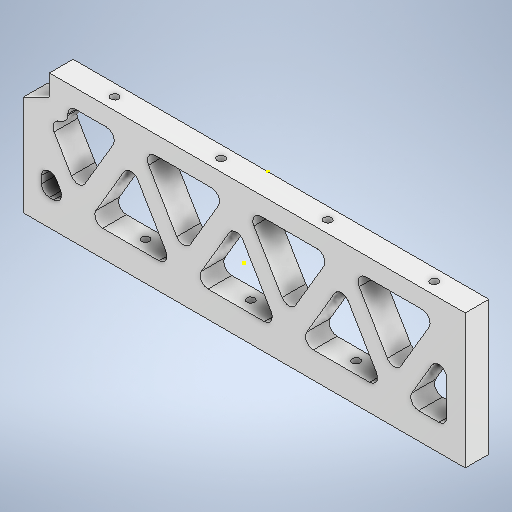
# Autodesk Inventor part: RightTruss
Saved by Autodesk Inventor 2026.2 (Build 302298000, 298)
## iProperties
Created: 2026-04-01
Part Number: RightTruss
Material: ABS Plastic
Document SubType Name: Modeling
Designer: gaoet
Density: 1.06 g/cm^3
Appearance: Smooth - White
Author: gaoet
Autodesk Inventor part; units mm, degrees
ref_plane "YZ Plane" through (0, 0, 0) normal (1, 0, 0) x (0, 1, 0)
ref_plane "XZ Plane" through (0, 0, 0) normal (0, 1, 0) x (-1, 0, 0)
ref_plane "XY Plane" through (0, 0, 0) normal (0, 0, 1) x (1, 0, 0)
sketch "Sketch1" plane through (0, 0, 0) normal (0, 0, 1) x (1, 0, 0)
  line L0 (-84, -25.5) -> (84, -25.5)
  line L1 (84, -25.5) -> (84, 25.5)
  line L2 (84, 25.5) -> (-84, 25.5)
  line L3 (-84, 25.5) -> (-84, -25.5)
  line L4 (-84, -25.5) -> (84, 25.5) construction
  line L5 (84, -25.5) -> (-84, 25.5) construction
  line L6 (-84, 17.5) -> (-74, 17.5)
  line L7 (-74, 17.5) -> (-74, 25.5)
  point P0 (0, 0)
  dimension "d0" = 168
  dimension "d1" = 51
  dimension "d2" = 10
  dimension "d3" = 8
  constraints: 16 end point, 2 horizontal, 2 midpoint, 2 parallel, 2 perpendicular, 2 point on line
  measures "d0" distance of L2.end L1.end
  measures "d1" distance of L0.end L1.end
  measures "d2" distance of L6.start L6.end
  measures "d3" distance of L6.end L7.end
extrude "Extrusion1" add sketch "Sketch1" along normal blind 9 contours L3 L6 L7 L2 L1 L0
chamfer "Chamfer1" distance 10 distance2 5 1 edges at (-84, 17.5, 4.5) measured on face at (-77.3333, 17.5, 3)
sketch "Sketch2" plane through (-84, -25.5, 0) normal (0, -1, 0) x (1, 0, 0)
  line L0 (0, 0) -> (0, 9) projected
  line L1 (0, 0) -> (168, 0) projected
  point P0 (84, 0)
  point P1 (22, 4.5)
  point P2 (42, 4.5)
  point P3 (62, 4.5)
  point P4 (82, 4.5)
  point P5 (102, 4.5)
  point P6 (122, 4.5)
  point P7 (142, 4.5)
  point P8 (162, 4.5)
  dimension "d9" = 22
  dimension "d10" = 4.5
  dimension "d13" = 20
  constraints: 1 horizontal, 7 other
  measures "d9" distance from line of L0 point (22, 4.5)
  measures "d10" distance from line of L1 point (22, 4.5)
  measures "d13" distance of point (22, 4.5) point (42, 4.5)
hole "Hole1" at (-62, -25.5, 4.5) at (-42, -25.5, 4.5) at (-22, -25.5, 4.5) at (-2, -25.5, 4.5) at (18, -25.5, 4.5) at (38, -25.5, 4.5) at (58, -25.5, 4.5) direction (0, 1, 0) diameter 3 depth 10
sketch "Sketch3" plane through (0, 0, 9) normal (0, 0, 1) x (1, 0, 0)
  line L0 (-63.5, -15.5) -> (-60.5, -15.5) projected
  line L1 (-84, 12.5) -> (-84, -25.5) projected
  line L2 (-84, -15.5) -> (84, -15.5)
  line L3 (84, -25.5) -> (84, 25.5) projected
  line L4 (-84, 12.5) -> (-74, 17.5) projected
  line L5 (-84, 12.5) -> (-84, -25.5) projected
  line L6 (-84, -25.5) -> (84, -25.5) projected
  line L7 (84, -25.5) -> (84, 25.5) projected
  line L8 (84, 25.5) -> (-74, 25.5) projected
  line L9 (-74, 25.5) -> (-74, 17.5) projected
  line L10 (-67, 18.5) -> (77, 18.5)
  line L11 (77, 18.5) -> (77, -18.5)
  line L12 (77, -18.5) -> (-77, -18.5)
  line L13 (-77, -18.5) -> (-77, 8.1738)
  line L14 (-77, 8.1738) -> (-67, 13.1738)
  line L15 (-67, 13.1738) -> (-67, 18.5)
  line L16 (77, 18.5) -> (56.9904, -15.5) construction
  line L17 (36.9807, 18.5) -> (56.9904, -15.5) construction
  line L18 (16.9711, -15.5) -> (36.9807, 18.5) construction
  line L19 (-3.0386, 18.5) -> (16.9711, -15.5) construction
  line L20 (-23.0482, -15.5) -> (-3.0386, 18.5) construction
  line L21 (-23.0482, -15.5) -> (-43.0579, 18.5) construction
  line L22 (-63.0675, -15.5) -> (-43.0579, 18.5) construction
  line L23 (-77, 8.1738) -> (-63.0675, -15.5) construction
  line L24 (-63.5, -15.5) -> (-60.5, -15.5) projected
  line L25 (-63.0675, -15.5) -> (-83.0772, 18.5) construction
  line L26 (-77, 1.2732) -> (-67.1287, -15.5)
  line L27 (-73.8622, 9.7427) -> (-59.0064, -15.5)
  line L28 (-47.119, 18.5) -> (-67.1287, -15.5)
  line L29 (-38.9968, 18.5) -> (-59.0064, -15.5)
  line L30 (-47.119, 18.5) -> (-27.1094, -15.5)
  line L31 (-38.9968, 18.5) -> (-18.9871, -15.5)
  line L32 (-7.0997, 18.5) -> (-27.1094, -15.5)
  line L33 (-18.9871, -15.5) -> (1.0225, 18.5)
  line L34 (-7.0997, 18.5) -> (12.9099, -15.5)
  line L35 (1.0225, 18.5) -> (21.0322, -15.5)
  line L36 (12.9099, -15.5) -> (32.9196, 18.5)
  line L37 (41.0418, 18.5) -> (61.0515, -15.5)
  line L38 (77, 11.5994) -> (61.0515, -15.5)
  line L39 (32.9196, 18.5) -> (52.9292, -15.5)
  line L40 (41.0418, 18.5) -> (21.0322, -15.5)
  line L41 (72.9389, 18.5) -> (52.9292, -15.5)
  point P0 (0, 0)
  point P1 (-73.0724, 1.5)
  point P2 (-72.0643, -7.1134)
  point P3 (26.9759, 1.5)
  point P4 (77, -15.5)
  point P5 (-3.0386, 11.5994)
  point P6 (56.9904, -8.5994)
  point P7 (36.9807, 11.5994)
  point P8 (16.9711, -8.5994)
  point P9 (-23.0482, -8.5994)
  point P10 (-43.0579, 11.5994)
  point P11 (-77, -15.5)
  point P12 (-63.0675, -8.5994)
  dimension "d25" = 7
  dimension "d30" = 3.5
  dimension "d31" = 3.5
  dimension "d32" = 3.5
  dimension "d33" = 3.5
  dimension "d34" = 3.5
  dimension "d35" = 3.5
  dimension "d36" = 3.5
  dimension "d37" = 3.5
  dimension "d38" = 3.5
  dimension "d39" = 3.5
  dimension "d40" = 3.5
  dimension "d41" = 3.5
  dimension "d42" = 3.5
  dimension "d43" = 3.5
  dimension "d44" = 3.5
  dimension "d46" = 3.5
  constraints: 60 end point, 16 parallel, 7 equal length, 7 point on line, 3 midpoint, 1 collinear, 1 horizontal, 1 horizontal alignment, 47 other
  measures "d30" distance from line of point (-73.072, 1.5) L27
  measures "d31" distance from line of point (-72.064, -7.113) L23
  measures "d32" distance between parallel lines of L22 L28
  measures "d33" distance between parallel lines of L29 L22
  measures "d34" distance between parallel lines of L30 L21
  measures "d35" distance between parallel lines of L21 L31
  measures "d36" distance between parallel lines of L20 L32
  measures "d37" distance between parallel lines of L20 L33
  measures "d38" distance between parallel lines of L19 L34
  measures "d39" distance between parallel lines of L19 L35
  measures "d40" distance from line of point (26.976, 1.5) L36
  measures "d41" distance between parallel lines of L40 L18
  measures "d42" distance between parallel lines of L17 L39
  measures "d43" distance between parallel lines of L17 L37
  measures "d44" distance between parallel lines of L16 L38
  measures "d46" distance between parallel lines of L16 L41
extrude "Extrusion2" cut sketch "Sketch3" against normal through all contours L2 L13 L26 | L29 L30 L2 | L27 L14 L15 L10 L28 | L33 L34 L2 | L31 L10 L32 | L2 L38 L11 | L40 L39 L2 | L35 L10 L36 | L37 L10 L41
fillet "Fillet1" radius 3 29 edges at (-67, 18.5, 4.5) (-67, 13.1738, 4.5) (-73.8622, 9.7427, 4.5) (-77, -15.5, 4.5) (-67.1287, -15.5, 4.5) (-43.0579, 11.5994, 4.5) (-47.119, 18.5, 4.5) (-63.0675, -8.5994, 4.5) (-59.0064, -15.5, 4.5) (-27.1094, -15.5, 4.5) (-23.0482, -8.5994, 4.5) (-38.9968, 18.5, 4.5) (-7.0997, 18.5, 4.5) (-18.9871, -15.5, 4.5) (-3.0386, 11.5994, 4.5) (12.9099, -15.5, 4.5) (16.9711, -8.5994, 4.5) (1.0225, 18.5, 4.5) (61.0515, -15.5, 4.5) (77, 11.5994, 4.5) (72.9389, 18.5, 4.5) (41.0418, 18.5, 4.5) (32.9196, 18.5, 4.5) (36.9807, 11.5994, 4.5) (21.0322, -15.5, 4.5) (52.9292, -15.5, 4.5) (56.9904, -8.5994, 4.5) (-77, 1.2732, 4.5) (77, -15.5, 4.5)
sketch "Sketch4" plane through (-74, 25.5, 0) normal (0, 1, 0) x (1, 0, 0)
  point P0 (74, 0)
sketch "Sketch5" plane through (-74, 25.5, 0) normal (0, 1, 0) x (1, 0, 0)
  line L0 (158, 0) -> (158, -9) projected
  line L1 (0, 0) -> (0, -9) projected
  line L2 (158, 0) -> (0, 0) projected
  line L3 (-10, 0) -> (-10, -9) projected
  point P0 (74, 0)
  point P1 (20.2499, -4.5)
  point P2 (60.7499, -4.5)
  point P3 (101.2499, -4.5)
  point P4 (141.7499, -4.5)
  point P5 (0, -4.5)
  dimension "d50" = 158
  dimension "d52" = 40.5
  dimension "d53" = 40.5
  dimension "d54" = 40.5
  dimension "d55" = 4.5
  dimension "d79" = 20.2499
  constraints: 3 horizontal alignment, 1 midpoint
  measures "d50" distance between parallel lines of L0 L1
  measures "d52" distance of point (60.75, -4.5) point (20.25, -4.5)
  measures "d53" distance of point (101.25, -4.5) point (60.75, -4.5)
  measures "d54" distance of point (141.75, -4.5) point (101.25, -4.5)
  measures "d55" distance from line of L2 point (20.25, -4.5)
  measures "d79" distance of point (0, -4.5) point (20.25, -4.5)
hole "Hole2" at (-13.2501, 25.5, 4.5) at (-53.7501, 25.5, 4.5) at (27.2499, 25.5, 4.5) at (67.7499, 25.5, 4.5) direction (0, -1, 0) diameter 3 depth 10
sketch "Sketch6" plane through (0, 0, 9) normal (0, 0, 1) x (1, 0, 0)
  point P0 (0, 0)
sketch "Sketch8" plane through (-74, 25.5, 0) normal (0, 1, 0) x (1, 0, 0)
  circle A0 centre (141.7499, -4.5) radius 1.5 projected
  circle A1 centre (101.2499, -4.5) radius 1.5 projected
  circle A2 centre (20.2499, -4.5) radius 1.5 projected
  circle A3 centre (60.7499, -4.5) radius 1.5 projected
  line L0 (158, 0) -> (0, 0) projected
  line L1 (0, 0) -> (0, -9) projected
  line L2 (158, -9) -> (0, -9) projected
  line L3 (158, 0) -> (158, -9) projected
  line L4 (154, 0) -> (154, -9)
  point P0 (74, 0)
  point P1 (158, -4.5)
  point P2 (154, -4.5)
  dimension "d67" = 4
  constraints: 2 end point, 2 midpoint, 2 point on line, 1 perpendicular, 1 vertical
  measures "d67" distance of point (158, -4.5) point (154, -4.5)
extrude "Extrusion4" [suppressed]
sketch "Sketch9" plane through (-84, -25.5, 0) normal (0, -1, 0) x (1, 0, 0)
  circle A0 centre (142, 4.5) radius 1.5 projected
  circle A1 centre (122, 4.5) radius 1.5 projected
  circle A2 centre (102, 4.5) radius 1.5 projected
  circle A3 centre (82, 4.5) radius 1.5 projected
  circle A4 centre (62, 4.5) radius 1.5 projected
  circle A5 centre (42, 4.5) radius 1.5 projected
  circle A6 centre (22, 4.5) radius 1.5 projected
  line L0 (0, 0) -> (168, 0) projected
  line L1 (168, 0) -> (168, 9) projected
  line L2 (0, 9) -> (168, 9) projected
  line L3 (0, 0) -> (0, 9) projected
  point P0 (84, 0)
  point P1 (162, 4.5)
  dimension "d70" = 20
  constraints: 1 horizontal alignment
  measures "d70" distance of point (162, 4.5) A0.centre
hole "Hole3" at (78, -25.5, 4.5) direction (0, 1, 0) diameter 3 depth 10
equation "\"d30\" = 0.5 * d25"
equation "\"d31\" = 0.5 * d25"
equation "\"d32\" = 0.5 * d25"
equation "\"d33\" = 0.5 * d25"
equation "\"d34\" = 0.5 * d25"
equation "\"d35\" = 0.5 * d25"
equation "\"d36\" = 0.5 * d25"
equation "\"d37\" = 0.5 * d25"
equation "\"d38\" = 0.5 * d25"
equation "\"d39\" = 0.5 * d25"
equation "\"d40\" = 0.5 * d25"
equation "\"d41\" = 0.5 * d25"
equation "\"d42\" = 0.5 * d25"
equation "\"d43\" = 0.5 * d25"
equation "\"d44\" = 0.5 * d25"
equation "\"d46\" = 0.5 * d25"
equation "\"d53\" = d52"
equation "\"d54\" = d53"
equation "\"d51\" = 0.125 * d50"
body "Solid1"
